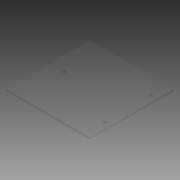
# Autodesk Inventor part: base
Saved by Autodesk Inventor 2012 SP1 (Build 160190100, 190)
## iProperties
Created: 2014-12-30
Part Number: base
Material: Default
Document SubType Name: Modeling
Designer: PRINCIPAL
Density: 1 g/cm^3
Author: PRINCIPAL
Autodesk Inventor part; units mm, degrees
ref_plane "YZ Plane" through (0, 0, 0) normal (1, 0, 0) x (0, 1, 0)
ref_plane "XZ Plane" through (0, 0, 0) normal (0, 1, 0) x (-1, 0, 0)
ref_plane "XY Plane" through (0, 0, 0) normal (0, 0, 1) x (1, 0, 0)
sketch "Boceto1" plane through (0, 0, 0) normal (0, 0, 1) x (1, 0, 0)
  line L0 (0, 0) -> (200, 0)
  line L1 (200, 0) -> (200, -200)
  line L2 (200, -200) -> (0, -200)
  line L3 (0, -200) -> (0, 0)
  dimension "d0" = 200
  dimension "d1" = 200
  constraints: 8 end point, 2 parallel, 1 horizontal, 1 perpendicular
  measures "d0" distance of L1.end L2.end
  measures "d1" distance of L0.end L1.end
extrude "Extrusión1" add sketch "Boceto1" along normal blind 5
sketch "Boceto2" plane through (0, 0, 5) normal (0, 0, 1) x (1, 0, 0)
  line L0 (200, 0) -> (200, -200) projected
  line L1 (200, -200) -> (0, -200) projected
  circle A0 centre (186, -40.5) radius 4
  circle A1 centre (186, -150.5) radius 4
  circle A2 centre (34.5, -95.5) radius 4
  dimension "d4" = 8
  dimension "d5" = 8
  dimension "d6" = 8
  dimension "d7" = 49.5
  dimension "d8" = 14
  dimension "d9" = 14
  dimension "d16" = 165.5
  dimension "d17" = 110
  dimension "d18" = 104.5
  constraints: 3 centre point
  measures "d4" diameter of A2
  measures "d5" diameter of A0
  measures "d6" diameter of A1
  measures "d7" distance from line of A1.centre L1
  measures "d8" distance from line of A1.centre L0
  measures "d9" distance from line of L0 A0.centre
  measures "d16" distance from line of L0 A2.centre
  measures "d17" distance of A0.centre A1.centre
  measures "d18" distance from line of L1 A2.centre
extrude "Extrusión2" cut sketch "Boceto2" against normal blind 5
